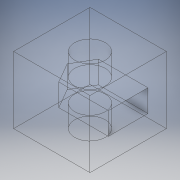
# Autodesk Inventor part: halfinchNUT
Saved by Autodesk Inventor 2018 (Build 220112000, 112)
## iProperties
Created: 2017-06-15
Part Number: halfinchNUT
Material: Generic
Document SubType Name: Modeling
Designer: Soichi
Density: 1 g/cm^3
Appearance: Default
Author: Soichi
Autodesk Inventor part; units mm, degrees
ref_plane "YZ Plane" through (0, 0, 0) normal (1, 0, 0) x (0, 1, 0)
ref_plane "XZ Plane" through (0, 0, 0) normal (0, 1, 0) x (-1, 0, 0)
sketch "Sketch1" plane through (0, 0, 0) normal (0, 0, 1) x (1, 0, 0)
  line L0 (0, -10.9985) -> (-9.525, -5.4993)
  line L1 (-9.525, -5.4993) -> (-9.525, 5.4993)
  line L2 (-9.525, 5.4993) -> (0, 10.9985)
  line L3 (0, 10.9985) -> (9.525, 5.4993)
  line L4 (9.525, 5.4993) -> (9.525, -5.4993)
  line L5 (9.525, -5.4993) -> (0, -10.9985)
  point P0 (0, 0)
  point P1 (0, 0)
  dimension "d0" = 19.05
  dimension "d1" = 21.9971
  constraints: 12 end point, 1 coincident, 1 vertical, 13 other
  measures "d0" distance between parallel lines of L4 L1
  measures "d1" distance of L0.start L2.end
sketch "Sketch2" plane through (0, 0, 0) normal (0, 0, 1) x (1, 0, 0)
  line L0 (-19.05, -19.05) -> (-19.05, 19.05)
  line L1 (-19.05, 19.05) -> (19.05, 19.05)
  line L2 (19.05, 19.05) -> (19.05, -19.05)
  line L3 (19.05, -19.05) -> (-19.05, -19.05)
  circle A0 centre (0, 0) radius 6.35 construction
  circle A1 centre (0, 0) radius 6.35 construction
  line L4 (0, -10.9985) -> (-9.525, -5.4993) construction
  line L5 (-9.525, -5.4993) -> (-9.525, 5.4993) construction
  line L6 (-9.525, 5.4993) -> (0, 10.9985) construction
  line L7 (0, 10.9985) -> (9.525, 5.4993) construction
  line L8 (9.525, 5.4993) -> (9.525, -5.4993) construction
  line L9 (9.525, -5.4993) -> (0, -10.9985) construction
  line L10 (0, 11.4027) -> (-9.875, 5.7013)
  line L11 (-9.875, 5.7013) -> (-9.875, -5.7013) construction
  line L12 (-9.875, -5.7013) -> (0, -11.4027) construction
  line L13 (0, -11.4027) -> (9.875, -5.7013) construction
  line L14 (9.875, -5.7013) -> (9.875, 5.7013) construction
  line L15 (9.875, 5.7013) -> (0, 11.4027)
  line L16 (-9.875, 5.7013) -> (-9.875, -19.05)
  line L17 (9.875, 5.7013) -> (9.875, -19.05)
  dimension "d11" = 38.1
  dimension "d12" = 0.35
  constraints: 24 end point, 3 point on line, 1 coincident, 1 horizontal, 1 perpendicular, 14 other
  measures "d11" distance of L2.end L0.start
  measures "d12" distance between parallel lines of L6 L10
extrude "Extrusion2" add sketch "Sketch2" along normal blind 11.1125 contours L0 L1 L2 L3 L17 L15 L10 L16
extrude "Extrusion4" add sketch "Sketch2" against normal blind 11.1125
ref_plane "Work Plane1" through (0, 0, 5.5563) normal (0, 0, 1) x (1, 0, 0)
mirror "Mirror1" about plane through (0, 0, 5.5563) normal (0, 0, 1) of "Extrusion4"
sketch "Sketch4" plane through (0, 0, -11.1125) normal (0, 0, -1) x (-1, 0, 0)
  point P0 (0, 0)
hole "Hole2" at (0, 0, -11.1125) direction (0, 0, 1) diameter 15.24 end through all
equation "\"d11\" = 2 * d0"
body "Solid1"
